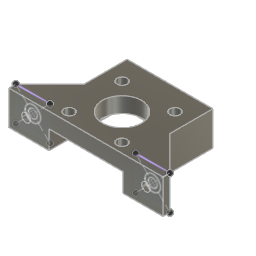
Z Axis Motor Mount (Autodesk Fusion 360 design; units mm, degrees)
Autodesk Fusion 360 part; units mm, degrees
note: some values were not read from the file. Set by a fixed rule: which sketch regions a step uses.
sketch "Sketch1" plane through (0, 0, 0) normal (0, 0, 1) x (1, 0, 0)
  line L0 (45.1, -24.6) -> (-45.1, -24.6)
  line L1 (-45.1, -24.6) -> (-45.1, 24.6)
  line L2 (-45.1, 24.6) -> (45.1, 24.6)
  line L3 (45.1, 24.6) -> (45.1, -24.6)
  line L4 (45.1, -24.6) -> (-45.1, 24.6) construction
  line L5 (-45.1, -24.6) -> (45.1, 24.6) construction
  dimension "d1" = 90.2
  dimension "d2" = 49.2
  constraint perpendicular L0 L1
  constraint parallel L0 L2
  constraint parallel L1 L3
  constraint horizontal L0
  constraint coincident L4 origin
  constraint coincident L5 origin
  measures "d1" distance of L1.end L2.end
  measures "d2" distance of L0.end L1.end L0.start
  measures "d5" distance of L0.start
extrude "Extrude1" add sketch "Sketch1" along normal blind 20
sketch "Sketch2" plane through (0, 0, 0) normal (0, 0, -1) x (-1, 0, 0)
  line L0 (40.1, -22.1) -> (40.1, 22.1)
  line L1 (40.1, 22.1) -> (-40.1, 22.1)
  line L2 (-40.1, 22.1) -> (-40.1, -22.1)
  line L3 (21.6, -24.6) -> (-21.6, -24.6)
  line L4 (-21.6, -24.6) -> (-21.6, 18.6)
  line L5 (-21.6, 18.6) -> (21.6, 18.6)
  line L6 (21.6, 18.6) -> (21.6, -24.6)
  line L7 (45.1, 24.6) -> (-45.1, 24.6)
  line L8 (-45.1, 24.6) -> (-45.1, -24.6)
  line L9 (-45.1, -24.6) -> (45.1, -24.6)
  line L10 (45.1, -24.6) -> (45.1, 24.6)
  dimension "d5" = 43.2
  dimension "d6" = 43.2
  dimension "d73" = 21.6
  constraint horizontal L3
  constraint vertical L4
  constraint horizontal L5
  constraint vertical L6
  constraint coincident L3.start L9
  measures "d5" distance of L3.start L3.end
  measures "d6" distance of L3.start L5.end
  measures "d73" distance of origin L6
extrude "Extrude2" cut sketch "Sketch2" against normal blind 11 contours L3 L4 L5 L6 L9
sketch "Sketch3" plane through (0, 24.6, 0) normal (0, 1, 0) x (-1, 0, 0)
  line L0 (-45.1, 0) -> (45.1, 0)
  line L1 (45.1, 0) -> (45.1, 20)
  line L2 (45.1, 20) -> (-45.1, 20)
  line L3 (-45.1, 20) -> (-45.1, 0)
  line L4 (-45.1, 20) -> (-25.1, 20)
  line L5 (-25.1, 20) -> (-25.1, 0)
  line L6 (-25.1, 0) -> (-45.1, 0)
  line L7 (-45.1, 0) -> (-45.1, 20)
  line L8 (45.1, 20) -> (25.1, 20)
  line L9 (25.1, 20) -> (25.1, 0)
  line L10 (25.1, 0) -> (45.1, 0)
  line L11 (45.1, 0) -> (45.1, 20)
  dimension "d9" = 20
  dimension "d10" = 20
  constraint horizontal L4
  constraint vertical L5
  constraint horizontal L6
  constraint vertical L7
  constraint coincident L2.end L3.start
  constraint horizontal L8
  constraint vertical L9
  constraint horizontal L10
  constraint vertical L11
  constraint coincident L1.end L2.start
  measures "d9" distance of L2.end L4.end
  measures "d10" distance of L1.end L8.end
extrude "Extrude3" cut sketch "Sketch3" against normal blind 45.2 contours L0 L2 L3 L4 L5 L6 L7 | L0 L1 L2 L8 L9 L10 L11
sketch "Sketch4" plane through (0, 0, 20) normal (0, 0, 1) x (-1, 0, 0)
  line L0 (25.1, -24.6) -> (25.1, 20.6)
  line L1 (25.1, 20.6) -> (45.1, 20.6)
  line L2 (45.1, 20.6) -> (45.1, 24.6)
  line L3 (45.1, 24.6) -> (-45.1, 24.6)
  line L4 (-45.1, 24.6) -> (-45.1, 20.6)
  line L5 (-45.1, 20.6) -> (-25.1, 20.6)
  line L6 (-25.1, 20.6) -> (-25.1, -24.6)
  line L7 (-25.1, -24.6) -> (25.1, -24.6)
  line L8 (25.1, 19) -> (-25.1, 19) construction
  line L9 (25.1, -12) -> (-25.1, -12) construction
  line L10 (15.5, -24.6) -> (15.5, 19) construction
  line L11 (-15.5, -24.6) -> (-15.5, 19) construction
  line L12 (15.5, -12) -> (15.5, -15) construction
  line L13 (15.5, -12) -> (15.5, -15) construction
  line L14 (0, -24.6) -> (0, 24.6) construction
  line L15 (-25.1, 3.5) -> (25.1, 3.5) construction
  circle A0 centre (15.5, -12) radius 1.7
  circle A1 centre (15.5, -12) radius 3
  circle A2 centre (-15.5, -12) radius 1.7
  circle A3 centre (-15.5, -12) radius 3
  circle A4 centre (-15.5, 19) radius 3
  circle A5 centre (-15.5, 19) radius 1.7
  circle A6 centre (15.5, 19) radius 3
  circle A7 centre (15.5, 19) radius 1.7
  dimension "d59" = 9.6
  dimension "d60" = 9.6
  dimension "d68" = 3.4
  dimension "d69" = 6
  dimension "d70" = 31
  dimension "d71" = 15.5
  constraint coincident L0 L8.start
  constraint coincident L6 L8.end
  constraint perpendicular L6 L8
  constraint coincident L0 L9.start
  constraint coincident L6 L9.end
  constraint perpendicular L6 L9
  constraint coincident L7 L10.start
  constraint coincident L8 L10.end
  constraint perpendicular L8 L10
  constraint coincident L7 L11.start
  constraint coincident L8 L11.end
  constraint perpendicular L8 L11
  constraint coincident L10 L12.end
  constraint coincident L9 L12.start
  constraint coincident L12.end L13.end
  constraint coincident L12.start L13.start
  constraint midpoint L7 L14.start
  constraint midpoint L3 L14.end
  constraint coincident L6 L15.start
  constraint coincident L0 L15.end
  constraint perpendicular L0 L15
  constraint concentric A0 A1
  constraint symmetric L14 A0 A2
  constraint symmetric L14 A1 A3
  constraint symmetric L15 A0 A7
  constraint symmetric L15 A1 A6
  constraint symmetric L15 A2 A5
  constraint symmetric L15 A3 A4
  measures "d59" distance of L6 L11
  measures "d60" distance of L0 L10
  measures "d68" diameter of A0
  measures "d69" diameter of A1
  measures "d70" distance of L8 L9
  measures "d71" distance of L9 L15
extrude "Extrude5" cut sketch "Sketch4" against normal blind 5 contours A0 | A1 | A2 | A3 | A4 | A5 | A6 | A7
extrude "Extrude4" cut sketch "Sketch4" against normal blind 9 from surface at -5.2 contours A0 | A2 | A5 | A7
sketch "Sketch5" plane through (0, -20.6, 0) normal (0, 1, 0) x (-1, 0, 0)
  line L0 (-45.1, 20) -> (-45.1, 0)
  line L1 (-45.1, 0) -> (-25.1, 0)
  line L2 (-25.1, 0) -> (-25.1, 20)
  line L3 (-25.1, 20) -> (-45.1, 0) construction
  line L4 (-45.1, 20) -> (-25.1, 0) construction
  circle A0 centre (-35.1, 10) radius 2.5
  circle A1 centre (-35.1, 10) radius 4.5
  line L5 (-25.1, 20) -> (-45.1, 20)
  dimension "d33" = 5
  dimension "d34" = 9
  constraint coincident L2.end L3.start
  constraint coincident L0.end L1.start
  constraint coincident L0.start L4.start
  constraint coincident L1.end L2.start
  constraint midpoint L3 A0.centre
  constraint concentric A0 A1
  measures "d33" diameter of A0
  measures "d34" diameter of A1
extrude "Extrude8" cut sketch "Sketch5" against normal blind 1 contours A0 | A1
extrude "Extrude7" cut sketch "Sketch5" against normal blind 4 contours A0
sketch "Sketch6" plane through (0, -20.6, 0) normal (0, 1, 0) x (-1, 0, 0)
  line L0 (45.1, 0) -> (45.1, 20)
  line L1 (25.1, 20) -> (25.1, 0)
  line L2 (25.1, 0) -> (45.1, 0)
  line L3 (25.1, 0) -> (45.1, 20) construction
  line L4 (25.1, 20) -> (45.1, 0) construction
  circle A0 centre (35.1, 10) radius 2.5
  circle A1 centre (35.1, 10) radius 4.5
  line L5 (45.1, 20) -> (25.1, 20)
  dimension "d39" = 5
  dimension "d40" = 9
  constraint coincident L1.end L2.start
  constraint coincident L0.end L3.end
  constraint coincident L1.start L4.start
  constraint coincident L0.start L2.end
  constraint midpoint L4 A0.centre
  constraint concentric A0 A1
  measures "d39" diameter of A0
  measures "d40" diameter of A1
extrude "Extrude10" cut sketch "Sketch6" against normal blind 1 contours A0 | A1
extrude "Extrude9" cut sketch "Sketch6" against normal blind 4 contours A0
sketch "Sketch7" plane through (0, 0, 20) normal (0, 0, 1) x (-1, 0, 0)
  line L0 (25.1, -24.6) -> (25.1, 20.6)
  line L1 (25.1, 20.6) -> (45.1, 20.6)
  line L2 (45.1, 20.6) -> (45.1, 24.6)
  line L3 (45.1, 24.6) -> (-45.1, 24.6)
  line L4 (-45.1, 24.6) -> (-45.1, 20.6)
  line L5 (-45.1, 20.6) -> (-25.1, 20.6)
  line L6 (-25.1, 20.6) -> (-25.1, -24.6)
  line L7 (-25.1, -24.6) -> (25.1, -24.6)
  line L8 (-25.1, 0.6) -> (25.1, 0.6) construction
  line L9 (45.1, 24.6) -> (-45.1, 24.6) construction
  line L10 (45.1, 20.6) -> (25.1, 0.6)
  line L11 (-25.1, 0.6) -> (-45.1, 20.6)
  line L12 (15.5, -12) -> (-15.5, 19) construction
  line L13 (15.5, 19) -> (-15.5, -12) construction
  line L14 (25.1, 2) -> (-25.1, 2) construction
  line L15 (-25.1, 0.5) -> (25.1, 0.5) construction
  line L16 (25.1, 3.5) -> (-25.1, 3.5) construction
  line L17 (0, 3.5) -> (0, 3.5473) construction
  circle A0 centre (15.5, -12) radius 3
  circle A1 centre (-15.5, 19) radius 3
  circle A2 centre (15.5, 19) radius 3
  circle A3 centre (-15.5, -12) radius 3
  circle A4 centre (0, 3.5) radius 11.5
  dimension "d50" = 24
  dimension "d64" = 22.6
  dimension "d65" = 1.5
  dimension "d66" = 1.5
  dimension "d74" = 23
  constraint coincident L6 L8.start
  constraint coincident L0 L8.end
  constraint perpendicular L0 L8
  constraint coincident L1.end L2.start
  constraint coincident L4.end L5.start
  constraint coincident L0 L14.start
  constraint coincident L6 L14.end
  constraint perpendicular L6 L14
  constraint coincident L6 L15.start
  constraint coincident L0 L15.end
  constraint perpendicular L0 L15
  constraint coincident L0 L16.start
  constraint coincident L6 L16.end
  constraint perpendicular L6 L16
  constraint perpendicular L15 L17
  constraint midpoint L16 L17.start
  constraint coincident L12.end A1.centre
  constraint coincident L13.start A2.centre
  constraint coincident L13.end A3.centre
  constraint coincident L12.start A0.centre
  constraint coincident L17.start A4.centre
  measures "d50" distance of L8 L9
  measures "d64" distance of L9 L14
  measures "d65" distance of L14 L15
  measures "d66" distance of L14 L16
  measures "d74" diameter of A4
extrude "Extrude13" cut sketch "Sketch7" against normal blind 9 contours A4
extrude "Extrude11" add sketch "Sketch7" against normal blind 4 contours L0 L1 L10 | L5 L6 L11
extrude "Extrude12" add sketch "Sketch7" along normal blind 4 from surface at -20 contours L0 L1 L10 | L5 L6 L11
chamfer "Chamfer1" distance 4 angle 45 2 edges at (21.6, 18.6, 5.5) (-21.6, 18.6, 5.5)
equation "d71 = d70 / 2"
equation "d73 = d5 / 2"
